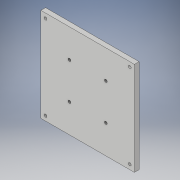
# Autodesk Inventor part: PhlangeForShop
Saved by Autodesk Inventor 2017 (Build 210142000, 142)
## iProperties
Created: 2017-07-07
Part Number: PhlangeForShop
Material: Generic
Document SubType Name: Modeling
Designer: sensor
Density: 1 g/cm^3
Appearance: Default
Author: sensor
Autodesk Inventor part; units mm, degrees
ref_plane "YZ Plane" through (0, 0, 0) normal (1, 0, 0) x (0, 1, 0)
ref_plane "XZ Plane" through (0, 0, 0) normal (0, 1, 0) x (-1, 0, 0)
ref_plane "XY Plane" through (0, 0, 0) normal (0, 0, 1) x (1, 0, 0)
sketch "Sketch1" plane through (0, 0, 0) normal (0, 0, 1) x (1, 0, 0)
  line L0 (0, 0) -> (200, 0)
  line L1 (200, 0) -> (200, 200)
  line L2 (200, 200) -> (0, 200)
  line L3 (0, 200) -> (0, 0)
  circle A0 centre (10, 190) radius 3
  circle A1 centre (190, 190) radius 3
  circle A2 centre (190, 10) radius 3
  circle A3 centre (10, 10) radius 3
  circle A4 centre (61.1091, 138.8909) radius 3
  circle A5 centre (61.1091, 61.1091) radius 3
  circle A6 centre (138.8909, 61.1091) radius 3
  circle A7 centre (138.8909, 138.8909) radius 3
  point P0 (164, 100)
  dimension "d1" = 200
  dimension "d5" = 10
  dimension "d6" = 10
  dimension "d7" = 10
  dimension "d8" = 10
  dimension "d9" = 6
  dimension "d10" = 6
  dimension "d11" = 10
  dimension "d12" = 10
  dimension "d14" = 10
  dimension "d15" = 6
  dimension "d16" = 6
  dimension "d17" = 6
  dimension "d18" = 6
  dimension "d19" = 6
  dimension "d20" = 6
  dimension "d42" = 200
  dimension "d43" = 10
  constraints: 8 centre point, 8 end point
  measures "d1" distance of L1.end L2.end
  measures "d5" distance from line of L2 A0.centre
  measures "d6" distance from line of L3 A0.centre
  measures "d7" distance from line of L1 A1.centre
  measures "d8" distance from line of L2 A1.centre
  measures "d9" diameter of A1
  measures "d10" diameter of A2
  measures "d11" distance from line of L1 A2.centre
  measures "d12" distance from line of L0 A2.centre
  measures "d14" distance from line of L0 A3.centre
  measures "d15" diameter of A3
  measures "d16" diameter of A0
  measures "d17" diameter of A7
  measures "d18" diameter of A4
  measures "d19" diameter of A5
  measures "d20" diameter of A6
  measures "d42" distance of L2.end L0.start
  measures "d43" distance from line of L3 A3.centre
extrude "Extrusion2" add sketch "Sketch1" along normal blind 10
thread "Thread1" size "M6x1" class "6H" standard "ANSI Metric M Profile" full length
thread "Thread2" size "M6x1" class "6H" standard "ANSI Metric M Profile" full length
thread "Thread3" size "M6x1" class "6H" standard "ANSI Metric M Profile" full length
thread "Thread4" size "M6x1" class "6H" standard "ANSI Metric M Profile" full length
body "Solid2"
